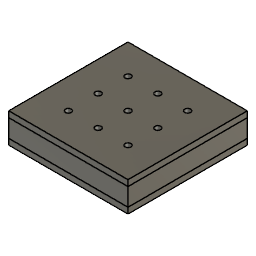
Probeta_Multicapa (Autodesk Fusion 360 design; units mm, degrees)
part number: 2026-04-24-10-34-14-119
Autodesk Fusion 360 part; units mm, degrees
note: some values were not read from the file. Chosen so that the rebuilt part matches the saved one: which bodies a step acts on; which face or edge a step refers to.
sketch "Boceto1" plane through (0, 0, 0) normal (0, 0, 1) x (1, 0, 0)
  line L0 (-40, -30) -> (20, -30)
  line L1 (20, -30) -> (20, 30)
  line L2 (20, 30) -> (-40, 30)
  line L3 (-40, 30) -> (-40, -30)
  constraint horizontal L0
  constraint vertical L1
  constraint horizontal L2
  constraint vertical L3
extrude "Extruir1" add sketch "Boceto1" along normal blind 15 makes body 1
hole "Agujero1" at (-25, -15, 15) direction (0, 0, -1) diameter 2.97 depth 3 tip angle 180 bodies 1
hole "Agujero2" at (-10, -15, 15) direction (0, 0, -1) diameter 2.97 depth 3 tip angle 180 bodies 1
hole "Agujero3" at (5, -15, 15) direction (0, 0, -1) diameter 2.97 depth 3 tip angle 180 bodies 1
hole "Agujero4" at (-25, 0, 15) direction (0, 0, -1) diameter 2.97 depth 3 tip angle 180 bodies 1
hole "Agujero5" at (-10, 0, 15) direction (0, 0, -1) diameter 2.97 depth 3 tip angle 180 bodies 1
hole "Agujero6" at (5, 0, 15) direction (0, 0, -1) diameter 2.97 depth 3 tip angle 180 bodies 1
hole "Agujero7" at (-25, 15, 15) direction (0, 0, -1) diameter 2.97 depth 3 tip angle 180 bodies 1
hole "Agujero8" at (-10, 15, 15) direction (0, 0, -1) diameter 2.97 depth 3 tip angle 180 bodies 1
hole "Agujero9" at (5, 15, 15) direction (0, 0, -1) diameter 2.97 depth 3 tip angle 180 bodies 1
hole "Agujero14" at (-35, -25, 0) direction (0, 0, 1) diameter 2.97 depth 3 tip angle 180 bodies 1
hole "Agujero15" at (15, 25, 0) direction (0, 0, 1) diameter 2.97 depth 3 tip angle 180 bodies 1
hole "Agujero16" at (-35, 25, 0) direction (0, 0, 1) diameter 2.97 depth 3 tip angle 180 bodies 1
hole "Agujero17" at (15, -25, 0) direction (0, 0, 1) diameter 2.97 depth 3 tip angle 180 bodies 1
ref_plane "PlanoDeObra3" through (0, 0, 3) normal (0, 0, 1) x (1, 0, 0)
ref_plane "PlanoDeObra4" through (0, 0, 12) normal (0, 0, 1) x (1, 0, 0)
split "Dividir1" by plane through (0, 0, 3) normal (0, 0, 1) and through (0, 0, 12) normal (0, 0, 1) bodies 1 makes body 2 at (-40, 10, 9) makes body 3 at (-35.4936, -0.037, 15)
ref_plane "PlanoDeObra5" through (0, -27, 0) normal (0, 1, 0) x (0, 0, 1)
copy_body "CopiarPegarCuerpos1" bodies 2 makes body 4
sketch "Boceto2" plane through (0, 0, 3) normal (0, 0, 1) x (1, 0, 0)
  line L0 (20, 0) -> (-40, 0)
  line L1 (-40, 0) -> (-40, -0.45)
  line L2 (-40, -0.45) -> (20, -0.45)
  line L3 (20, -0.45) -> (20, 0)
  dimension "d93" = 60
  dimension "d94" = 0.45
  constraint horizontal L0
  constraint vertical L1
  constraint horizontal L2
  constraint vertical L3
  measures "d93" distance of L0.start L0.end
  measures "d94" distance of L0.start L2.end
sketch "Boceto3" plane through (0, 0, 3) normal (0, 0, 1) x (1, 0, 0)
  line L0 (20, -30) -> (-40, -30)
  line L1 (-40, -30) -> (-40, -29.55)
  line L2 (-40, -29.55) -> (20, -29.55)
  line L3 (20, -29.55) -> (20, -30)
  dimension "d95" = 60
  dimension "d96" = 0.45
  constraint horizontal L0
  constraint vertical L1
  constraint horizontal L2
  constraint vertical L3
  measures "d95" distance of L0.start L0.end
  measures "d96" distance of L0.start L2.end
extrude "Extruir2" add sketch "Boceto3" along normal blind 9 separate body makes body 5
sketch "Boceto4" plane through (0, 0, 12) normal (0, 0, 1) x (-1, 0, 0)
  line L0 (-20, -5.7441) -> (40, -5.7441)
  line L1 (40, -5.7441) -> (40, -5.2941)
  line L2 (40, -5.2941) -> (-20, -5.2941)
  line L3 (-20, -5.2941) -> (-20, -5.7441)
  line L4 (-20, 30) -> (-19.55, 30)
  line L5 (-19.55, 30) -> (-19.55, -30)
  line L6 (-19.55, -30) -> (-20, -30)
  line L7 (-20, -30) -> (-20, 30)
  line L8 (40, 30) -> (40.45, 30)
  line L9 (40.45, 30) -> (40.45, -30)
  line L10 (40.45, -30) -> (40, -30)
  line L11 (40, -30) -> (40, 30)
  dimension "d103" = 0.45
  dimension "d104" = 60
  dimension "d105" = 0.45
  dimension "d106" = 60
  constraint horizontal L4
  constraint vertical L5
  constraint horizontal L6
  constraint vertical L7
  constraint horizontal L8
  constraint vertical L9
  constraint horizontal L10
  constraint vertical L11
  measures "d103" distance of L4.start L4.end
  measures "d104" distance of L4.start L6.end
  measures "d105" distance of L8.start L8.end
  measures "d106" distance of L8.start L10.end
sketch "Boceto5" plane through (0, 0, 3) normal (0, 0, 1) x (1, 0, 0)
sketch "Boceto6" plane through (0, 0, 3) normal (0, 0, 1) x (1, 0, 0)
  line L0 (-40, -30) -> (-39.55, -30)
  line L1 (-39.55, -30) -> (-39.55, 30)
  line L2 (-39.55, 30) -> (-40, 30)
  line L3 (-40, 30) -> (-40, -30)
  dimension "d107" = 0.45
  dimension "d108" = 60
  constraint horizontal L0
  constraint vertical L1
  constraint horizontal L2
  constraint vertical L3
  measures "d107" distance of L0.start L0.end
  measures "d108" distance of L0.start L2.end
extrude "Extruir3" add sketch "Boceto6" along normal blind 9 separate body makes body 6
pattern_linear "Patrón R2" count 2 spacing 59.55 along (1, 0, 0) of bodies 6 makes body 7
pattern_linear "Patrón R3" count 35 spacing 1.7485 along (0, 1, 0) of bodies 5 makes body 8 at (0, -28.2515, 9) makes body 9 at (0, -26.5029, 9) makes body 10 at (0, -24.7544, 9) makes body 11 at (0, -23.0059, 9) makes body 12 at (0, -21.2574, 9) makes body 13 at (0, -19.5088, 9) makes body 14 at (0, -17.7603, 9) makes body 15 at (0, -16.0118, 9) makes body 16 at (0, -14.2632, 9) makes body 17 at (0, -12.5147, 9) makes body 18 at (0, -10.7662, 9) makes body 19 at (0, -9.0176, 9) makes body 20 at (0, -7.2691, 9) makes body 21 at (0, -5.5206, 9) makes body 22 at (0, -3.7721, 9) makes body 23 at (0, -2.0235, 9) makes body 24 at (0, -0.275, 9) makes body 25 at (0, 1.4735, 9) makes body 26 at (0, 3.2221, 9) makes body 27 at (0, 4.9706, 9) makes body 28 at (0, 6.7191, 9) makes body 29 at (0, 8.4676, 9) makes body 30 at (0, 10.2162, 9) makes body 31 at (0, 11.9647, 9) makes body 32 at (0, 13.7132, 9) makes body 33 at (0, 15.4618, 9) makes body 34 at (0, 17.2103, 9) makes body 35 at (0, 18.9588, 9) makes body 36 at (0, 20.7074, 9) makes body 37 at (0, 22.4559, 9) makes body 38 at (0, 24.2044, 9) makes body 39 at (0, 25.9529, 9) makes body 40 at (0, 27.7015, 9) makes body 41 at (0, 29.45, 9)
sketch "Boceto7" plane through (0, 0, 0) normal (0, 0, 1) x (1, 0, 0)
  circle A0 centre (-35, 25) radius 1.5
  dimension "d119" = 3
  measures "d119" diameter of A0
extrude "Extruir4" add sketch "Boceto7" along normal blind 3 separate body makes body 42
pattern_linear "Patrón R4" count 2 spacing 50 along (0, -1, 0) of bodies 42 makes body 43
pattern_linear "Patrón R5" count 2 spacing 50 along (1, 0, 0) of bodies 43 42 makes body 44 at (16.4981, 24.9252, 2) makes body 45 at (16.4981, -25.0748, 2)
sketch "Boceto8" plane through (0, 0, 3) normal (0, 0, 1) x (-1, 0, 0)
  circle A0 centre (-15, 25) radius 1.485
  circle A1 centre (35, -25) radius 1.485
  circle A2 centre (-15, -25) radius 1.485
  circle A3 centre (35, 25) radius 1.485
  line L0 (-20, -30) -> (40, -30)
  line L1 (40, -30) -> (40, 30)
  line L2 (40, 30) -> (-20, 30)
  line L3 (-20, 30) -> (-20, -30)
  circle A4 centre (-5, -15) radius 1.5
  dimension "d130" = 3
  measures "d130" diameter of A4
ref_plane "PlanoDeObra6" through (-10, 0, 15) normal (0, 0, 1) x (-1, 0, 0)
sketch "Boceto9" plane through (0, 0, 15) normal (0, 0, 1) x (1, 0, 0)
  circle A0 centre (5, -15) radius 1.5
  dimension "d132" = 3
  measures "d132" diameter of A0
extrude "Extruir5" add sketch "Boceto9" against normal blind 3 separate body makes body 46
pattern_linear "Patrón R6" count 3 spacing 15 along (-1, 0, 0) of bodies 46 makes body 47 at (-8.5019, -15.0748, 13) makes body 48 at (-23.5019, -15.0748, 13)
pattern_linear "Patrón R7" count 3 spacing 15 along (0, 1, 0) of bodies 46 47 48 makes body 49 at (6.4981, -0.0748, 13) makes body 50 at (6.4981, 14.9252, 13) makes body 51 at (-8.5019, -0.0748, 13) makes body 52 at (-8.5019, 14.9252, 13) makes body 53 at (-23.5019, -0.0748, 13) makes body 54 at (-23.5019, 14.9252, 13)
combine "Combinar1" operation add target body 41 tool bodies 40 39 38 37 36 34 33 35 32 31 30 29 28 27 26 25 24 23 22 21 20 19 18 17 16 15 14 13 12 11 10 9 8 7 6 5
hidden bodies 4 41 42 43 44 45 46 47 48 49 50 51 52 53 54
named bodies: "Cerebro", "Craneo", "Cuero_Cabelludo"
